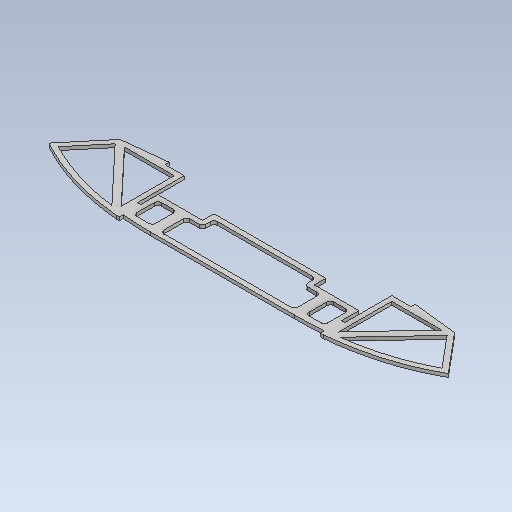
# Autodesk Inventor part: bulkhead_F1
Saved by Autodesk Inventor 2020.3 (Build 243373000, 373)
## iProperties
Created: 2020-05-22
Part Number: bulkhead_F1
Material: Generic
Document SubType Name: Modeling
Designer: kardo
Density: 1 g/cm^3
Appearance: Default
Mass: 4.97836 g
Surface Area: 76.7453 cm^2
Volume: 4.97836 cm^3
Author: kardo
Autodesk Inventor part; units mm, degrees
ref_plane "YZ Plane" through (0, 0, 0) normal (1, 0, 0) x (0, 1, 0)
ref_plane "XZ Plane" through (0, 0, 0) normal (0, 1, 0) x (-1, 0, 0)
ref_plane "XY Plane" through (0, 0, 0) normal (0, 0, 1) x (1, 0, 0)
derived "base_sketch.ipt"
sketch "bulkhead_F1" plane through (0, 56.1, 0) normal (0, 1, 0) x (-1, 0, 0)
  line L0 (19.176, 46.818) -> (62.322, 46.818)
  line L1 (-34.5168, 0) -> (-57.528, 27.54)
  line L2 (-11.5056, -2.4868) -> (-34.5168, 0)
  line L3 (-11.5056, 0) -> (-11.5056, -2.4868)
  line L4 (0, 0) -> (-11.5056, 0)
  line L5 (62.322, 46.818) -> (62.322, 13.529)
  line L6 (28.764, 19.935) -> (28.764, 13.529)
  line L7 (-38.1199, 4.3123) -> (-11.5056, 1.4361)
  line L8 (-11.5056, 1.4361) -> (-11.5056, 3.9229)
  line L9 (-11.5056, 3.9229) -> (0, 3.9229)
  line L10 (0, 3.9229) -> (0, 21.6458)
  line L11 (0, 21.6458) -> (28.764, 21.6458)
  line L12 (28.764, 21.6458) -> (28.764, 14.7544)
  line L13 (28.764, 14.7544) -> (62.322, 14.7544)
  line L14 (62.322, 43.2359) -> (19.176, 43.2359)
  line L15 (-57.528, 27.54) -> (-38.1199, 4.3123)
  line L16 (0, 45.9) -> (0, 44.8052) construction
  line L17 (-19.176, 42.5952) -> (-19.176, 41.8654) construction
  line L18 (-38.352, 36.72) -> (-38.352, 36.3551) construction
  line L19 (0, 19.935) -> (0, 0)
  line L20 (0, 44.8052) -> (0, 42.3179)
  spline S0 degree 4 poles (-57.528, 27.54) (-46.0483, 34.2051) (-30.6129, 40.5281) (-11.2214, 45.0414) (8.3201, 46.818) (15.5662, 46.818) (19.176, 46.818) knots 0 0 0 0 0 0.630279 0.815816 1 1 1 1 1
  spline S1 degree 3 poles (-57.528, 27.54) (-39.1506, 37.8756) (-19.5945, 42.9173) (0, 44.8052) knots 0 0 0 0 1 1 1 1
  spline S2 degree 2 poles (0, 42.3179) (9.5715, 43.2359) (19.176, 43.2359) knots 0 0 0 1 1 1
  line L21 (0, 35.7) -> (-57.528, 27.54) construction
  point P0 (0, 3.9229)
  point P1 (0, 14.7544)
  point P2 (0, 44.0613)
ref_plane "bulkhead_F1_plane" through (0, 56.1, 0) normal (0, 1, 0) x (-1, 0, 0)
sketch "Sketch2" plane through (0, 56.1, 0) normal (0, 1, 0) x (-1, 0, 0)
  spline S0 degree 2 poles (0, 42.3179) (9.5715, 43.2359) (19.176, 43.2359) knots 0 0 0 1 1 1 projected
  line L0 (62.322, 43.2359) -> (19.176, 43.2359) projected
  line L1 (62.322, 46.818) -> (62.322, 13.529) projected
  line L2 (28.764, 14.7544) -> (62.322, 14.7544) projected
  line L3 (28.764, 21.6458) -> (28.764, 14.7544) projected
  line L4 (0, 21.6458) -> (28.764, 21.6458) projected
  line L5 (0, 3.9229) -> (0, 21.6458) projected
  line L6 (-11.5056, 3.9229) -> (0, 3.9229) projected
  line L7 (-11.5056, 1.4361) -> (-11.5056, 3.9229) projected
  line L8 (-38.1199, 4.3123) -> (-11.5056, 1.4361) projected
  line L9 (-57.528, 27.54) -> (-38.1199, 4.3123) projected
  spline S1 degree 3 poles (-57.528, 27.54) (-39.1506, 37.8756) (-19.5945, 42.9173) (0, 44.8052) knots 0 0 0 0 1 1 1 1 projected
  line L10 (-52.8779, 26.6535) -> (-37.3404, 8.0581)
  line L11 (-37.3404, 8.0581) -> (-6.2686, 41.0642)
  line L12 (-32.9155, 6.9229) -> (-3, 38.7007)
  line L13 (-3, 38.7007) -> (-3, 6.9229)
  line L14 (-3, 6.9229) -> (-32.9155, 6.9229)
  line L15 (0, 21.6458) -> (0, 31.9819)
  line L16 (0, 31.9819) -> (2, 31.9819)
  line L17 (2, 31.9819) -> (2, 21.6458)
  line L18 (16.176, 37.3179) -> (16.176, 26.6458)
  line L19 (14.176, 24.6458) -> (7, 24.6458)
  line L20 (5, 26.6458) -> (5, 37.3179)
  line L21 (7, 39.3179) -> (14.176, 39.3179)
  line L22 (22.176, 38.2359) -> (22.176, 26.6458)
  line L23 (24.176, 24.6458) -> (29.764, 24.6458)
  line L24 (31.764, 22.6458) -> (31.764, 19.7544)
  line L25 (33.764, 17.7544) -> (62.322, 17.7544)
  line L26 (24.176, 40.2359) -> (62.322, 40.2359)
  spline S2 degree 2 poles (-52.8779, 26.6535) (-30.8463, 37.9763) (-6.2686, 41.0642) knots 0 0 0 1 1 1
  line L27 (-6.2686, 41.0642) -> (-6.6684, 44.0374) construction
  line L28 (-30.2098, 35.9176) -> (-31.0831, 38.7876) construction
  line L29 (-52.8779, 26.6535) -> (-54.2725, 29.3096) construction
  line L30 (-52.8779, 26.6535) -> (-30.2098, 35.9176) construction
  line L31 (-30.2098, 35.9176) -> (-6.2686, 41.0642) construction
  line L32 (-38.1199, 4.3123) -> (0, 44.8052) construction
  arc A0 (14.176, 24.6458) -> (16.176, 26.6458) centre (14.176, 26.6458) ccw
  arc A1 (5, 26.6458) -> (7, 24.6458) centre (7, 26.6458) ccw
  arc A2 (7, 39.3179) -> (5, 37.3179) centre (7, 37.3179) ccw
  arc A3 (16.176, 37.3179) -> (14.176, 39.3179) centre (14.176, 37.3179) ccw
  arc A4 (24.176, 40.2359) -> (22.176, 38.2359) centre (24.176, 38.2359) ccw
  arc A5 (22.176, 26.6458) -> (24.176, 24.6458) centre (24.176, 26.6458) ccw
  arc A6 (31.764, 22.6458) -> (29.764, 24.6458) centre (29.764, 22.6458) ccw
  arc A7 (31.764, 19.7544) -> (33.764, 17.7544) centre (33.764, 19.7544) ccw
  line L33 (62.322, 43.2359) -> (62.322, 14.7544)
  line L34 (0, 44.8052) -> (0, 42.3179) projected
  line L35 (0, 44.8052) -> (2, 44.8052)
  line L36 (2, 44.8052) -> (2, 42.4997)
  line L37 (0, 42.3179) -> (0, 31.9819) construction
  point P0 (0, 0)
  point P1 (-57.528, 25.7972)
  point P2 (0, 44.0613)
  dimension "d1" = 3
  dimension "d2" = 3
  dimension "d3" = 3
  dimension "d4" = 4
  dimension "d5" = 2
  dimension "d6" = 3
  dimension "d7" = 3
  dimension "d8" = 3
  dimension "d9" = 3
  dimension "d10" = 3
  dimension "d11" = 3
  dimension "d12" = 3
  dimension "d13" = 3
  dimension "d14" = 3
  dimension "d15" = 3
  dimension "d16" = 2
  constraints: 54 end point, 16 point on circle, 16 tangent, 8 centre point, 8 parallel, 7 equal radius, 7 vertical, 4 equal length, 3 horizontal, 3 point on line, 2 perpendicular, 1 collinear, 13 other
  measures "d1" distance between parallel lines of L6 L14
  measures "d2" distance between parallel lines of L5 L13
  measures "d4" distance between parallel lines of L12 L11
  measures "d5" distance between parallel lines of L17 L15
  measures "d6" distance between parallel lines of L20 L17
  measures "d7" distance from line of L34.end L21
  measures "d8" distance between parallel lines of L4 L19
  measures "d9" distance from line of L0.end L18
  measures "d10" distance from line of L0.end L22
  measures "d11" distance between parallel lines of L2 L25
  measures "d12" distance between parallel lines of L3 L24
  measures "d13" distance between parallel lines of L4 L23
  measures "d14" distance between parallel lines of L0 L26
  measures "d15" distance of L10.start L29.end
  measures "d16" radius of A0
extrude "Extrusion1" add sketch "Sketch2" along normal blind 2 contours L34 L35 L36 S0 | S0 L0 L1 L26 A4 L22 A5 L23 A6 L24 A7 L25 L2 L3 L4 L17 L16 L15 L5 L6 L7 L8 L9 S1 L34
mirror "Mirror1" about plane through (-62.322, 56.1, 14.7544) normal (-1, 0, 0) of "Extrusion1"
equation "\"d5\" = stringer_thickness"
equation "\"d17\" = bulkhead_thickness"
equation "\"stringer_thickness\" = 2"
equation "\"bulkhead_thickness\" = 2"
body "Solid1"
